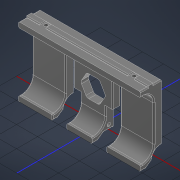
# Autodesk Inventor part: Skirt Front
Saved by Autodesk Inventor 2022.2 (Build 262287010, 287A)
## iProperties
Created: 2022-03-19
Part Number: Skirt Front
Material: ABS-Kunststoff
Document SubType Name: Modeling
Designer: sleib
Density: 1.06 g/cm^3
Appearance: Glatt - Schwarz
Author: sleib
Autodesk Inventor part; units mm, degrees
ref_plane "YZ Plane" through (0, 0, 0) normal (1, 0, 0) x (0, 1, 0)
ref_plane "XZ Plane" through (0, 0, 0) normal (0, 1, 0) x (-1, 0, 0)
ref_plane "XY Plane" through (0, 0, 0) normal (0, 0, 1) x (1, 0, 0)
sketch "Skirt" plane through (0, 0, 0) normal (0, 0, 1) x (1, 0, 0)
  line L0 (33, 20) -> (-33, 20) construction
  line L1 (-33, 20) -> (-33, 0) construction
  line L2 (-33, 0) -> (33, 0) construction
  line L3 (33, 0) -> (33, 20) construction
  line L4 (0, 20) -> (0, 0) construction
  line L5 (33, 20) -> (28, 20)
  line L6 (-33, 20) -> (-28, 20)
  line L7 (33, 20) -> (33, 13)
  line L8 (33, 0) -> (33, 7)
  line L9 (33, 13) -> (34, 13)
  line L10 (33, 7) -> (34, 7)
  line L11 (34, 7) -> (34, 13)
  line L12 (-29, 0) -> (-29, 9)
  line L13 (-29, 9) -> (-33, 14.7126)
  line L14 (-33, 20) -> (-33, 14.7126)
  line L15 (-28, 20) -> (-28, 18)
  line L16 (28, 20) -> (28, 18)
  arc A0 (17, 7) -> (28, 18) centre (17, 18) ccw
  arc A1 (-28, 18) -> (-17, 7) centre (-17, 18) ccw
  line L17 (17, 7) -> (-17, 7)
  line L18 (-29, 0) -> (33, 0)
  line L19 (33, 0.4) -> (32.6, 0)
  line L20 (-29, 0.4) -> (-28.6, 0)
  line L21 (33.2, 13) -> (34, 12.2)
  line L22 (34, 7.8002) -> (33.2, 7)
  point P0 (34, 10)
  point P1 (33, 10)
  dimension "d4" = 66
  dimension "d5" = 20
  dimension "d6" = 5
  dimension "d7" = 5
  dimension "d18" = 1
  dimension "d23" = 9
  dimension "d24" = 4
  dimension "d27" = 35
  dimension "d31" = 2
  dimension "d32" = 2
  dimension "d34" = 6
  dimension "d35" = 13
  dimension "d36" = 0.4
  dimension "d37" = 0.4
  dimension "d38" = 0.4
  dimension "d39" = 0.4
  dimension "d40" = 0.2
  dimension "d41" = 0.8
  dimension "d42" = 0.8002
  measures "d4" distance of L5.start L14.start
  measures "d5" distance of L8.start L5.start
  measures "d6" distance of L5.start L16.start
  measures "d7" distance of L14.start L15.start
  measures "d18" distance of L9.start L11.end
  measures "d23" distance of L12.start L12.end
  measures "d24" distance between parallel lines of L12 L14
  measures "d27" angle of L1 L13
  measures "d31" distance of L15.start L15.end
  measures "d32" distance of L16.start L16.end
  measures "d34" distance between parallel lines of L10 L9
  measures "d35" distance between parallel lines of L17 L0
  measures "d36" distance from line of L18 L19.start
  measures "d37" distance from line of L8 L19.end
  measures "d38" distance from line of L18 L20.start
  measures "d39" distance from line of L12 L20.end
  measures "d40" distance from line of L7 L21.start
  measures "d41" distance from line of L21.end L9
  measures "d42" distance from line of L10 L22.start
sketch "Skizze1" plane through (0, 0, 0) normal (1, 0, 0) x (0, 1, 0)
  circle A0 centre (-25, 4) radius 4 construction
  circle A1 centre (-25, 4) radius 1.7
  circle A2 centre (-25, 4) radius 3
  arc A3 (-20.4767, 0) -> (-29, 9) centre (-29.49, 0) ccw
  line L0 (33, 20) -> (-33, 20) construction
  line L1 (-33, 20) -> (-33, 0) construction
  line L2 (-33, 0) -> (33, 0) construction
  line L3 (33, 0) -> (33, 20) construction
  line L4 (0, 20) -> (0, 0) construction
  line L5 (33, 20) -> (28, 20)
  line L6 (-33, 20) -> (-28, 20)
  line L7 (33, 20) -> (33, 13)
  line L8 (33, 0) -> (33, 7)
  line L9 (33, 13) -> (34, 13)
  line L10 (33, 7) -> (34, 7)
  line L11 (34, 7) -> (34, 13)
  line L12 (-29, 0) -> (-29, 9)
  line L13 (-29, 9) -> (-33, 14.7126)
  line L14 (-33, 20) -> (-33, 14.7126)
  line L15 (-28, 20) -> (-28, 18)
  line L16 (28, 20) -> (28, 18)
  arc A4 (17, 7) -> (28, 18) centre (17, 18) ccw
  arc A5 (-28, 18) -> (-17, 7) centre (-17, 18) ccw
  line L17 (17, 7) -> (-17, 7)
  line L18 (-29, 0) -> (33, 0)
  line L19 (33, 0.4) -> (32.6, 0)
  line L20 (-29, 0.4) -> (-28.6, 0)
  line L21 (33.2, 13) -> (34, 12.2)
  line L22 (34, 7.8002) -> (33.2, 7)
  point P0 (-20.4767, 0)
  point P1 (-22.76, 5.9956)
  dimension "d43" = 8
  dimension "d44" = 3.4
  dimension "d80" = 6
  constraints: 4 centre point, 2 coincident, 2 point on circle, 1 tangent, 7 other
  measures "d43" diameter of A0
  measures "d44" diameter of A1
  measures "d80" diameter of A2
extrude "Extrusion1" add sketch "Skizze1" along normal mid plane 116 contours A3 L13 L14 L6 L15 A5 L17 A4 L16 L5 L7 L9 L21 L11 L22 L10 L8 L19 L18
sketch "Skizze2" plane through (58, 32.6, 0) normal (0, 0, -1) x (-1, 0, 0)
  line L0 (0, -65.6) -> (46, -65.6)
  line L1 (46, -65.6) -> (46, -40.6)
  line L2 (116, -65.6) -> (70, -65.6)
  line L3 (70, -65.6) -> (70, -40.6)
  line L4 (116, -65.6) -> (0, -65.6) projected
  line L5 (39.5, -40.6) -> (39.5, -15.6)
  line L6 (76.5, -40.6) -> (76.5, -15.6)
  line L7 (116, -15.6) -> (0, -15.6) projected
  line L8 (64, -22.2077) -> (70, -32.6)
  line L9 (70, -32.6) -> (64, -42.9923)
  line L10 (64, -42.9923) -> (52, -42.9923)
  line L11 (52, -42.9923) -> (46, -32.6)
  line L12 (46, -32.6) -> (52, -22.2077)
  line L13 (52, -22.2077) -> (64, -22.2077)
  line L14 (58, -15.6) -> (58, -65.6) construction
  line L15 (39.5, -40.6) -> (46, -40.6)
  line L16 (70, -40.6) -> (76.5, -40.6)
  line L17 (0, -15.6) -> (32, -15.6)
  line L18 (32, -15.6) -> (32, -65.6)
  line L19 (32, -65.6) -> (0, -65.6)
  line L20 (0, -65.6) -> (0, -15.6)
  line L21 (116, -15.6) -> (84, -15.6)
  line L22 (84, -15.6) -> (84, -65.6)
  line L23 (84, -65.6) -> (116, -65.6)
  line L24 (116, -65.6) -> (116, -15.6)
  point P0 (58, -32.6)
  point P1 (58, -32.6)
  point P2 (39.5, -15.6)
  point P3 (76.5, -15.6)
  dimension "d53" = 4
  dimension "d54" = 6.6077
  dimension "d55" = 24
  dimension "d56" = 37
  dimension "d78" = 25
  dimension "d79" = 7.5
  constraints: 46 end point, 7 horizontal, 4 parallel, 4 perpendicular, 3 point on line, 2 collinear, 2 midpoint, 1 coincident, 16 other
  measures "d53" distance from line of L1.end L11
  measures "d54" distance between parallel lines of L13 L7
  measures "d55" distance between parallel lines of L3 L1
  measures "d56" distance between parallel lines of L6 L5
  measures "d78" distance between parallel lines of L4 L15
  measures "d79" distance between parallel lines of L5 L18
extrude "Extrusion2" cut sketch "Skizze2" against normal through all contours L18 L7 L5 L15 L1 L0 | L3 L16 L6 L7 L22 L2 | L8 L9 L10 L11 L12 L13
extrude "Extrusion7" add sketch "Skizze1" along normal mid plane 24 contours A2 | A3 L18 L20 L12
fillet "Rundung1" radius 3 6 edges at (6, 10.3923, 3.5) (-6, 10.3923, 3.5) (-12, 0, 3.5) (-6, -10.3923, 3.5) (6, -10.3923, 3.5) (12, 0, 3.5)
sketch "Skizze3" plane through (58, 32.6, 0) normal (0, 0, -1) x (-1, 0, 0)
  line L0 (116, 0) -> (116, -53.0767) projected
  line L1 (116, 0) -> (0, 0) projected
  line L2 (0, -53.0767) -> (0, 0) projected
  line L3 (51.134, -41.4923) -> (46.866, -34.1) projected
  arc A0 (46.866, -31.1) -> (46.866, -34.1) centre (49.4641, -32.6) ccw projected
  line L4 (46.866, -31.1) -> (51.134, -23.7077) projected
  arc A1 (53.7321, -22.2077) -> (51.134, -23.7077) centre (53.7321, -25.2077) ccw projected
  line L5 (53.7321, -22.2077) -> (62.2679, -22.2077) projected
  arc A2 (64.866, -23.7077) -> (62.2679, -22.2077) centre (62.2679, -25.2077) ccw projected
  line L6 (64.866, -23.7077) -> (69.134, -31.1) projected
  arc A3 (69.134, -34.1) -> (69.134, -31.1) centre (66.5359, -32.6) ccw projected
  line L7 (69.134, -34.1) -> (64.866, -41.4923) projected
  arc A4 (62.2679, -42.9923) -> (64.866, -41.4923) centre (62.2679, -39.9923) ccw projected
  line L8 (62.2679, -42.9923) -> (53.7321, -42.9923) projected
  arc A5 (51.134, -41.4923) -> (53.7321, -42.9923) centre (53.7321, -39.9923) ccw projected
  line L9 (116, 1.4) -> (0, 1.4) projected
  line L10 (0, 0.6) -> (0, 1.4) projected
  line L11 (116, 0.6) -> (0, 0.6) projected
  line L12 (116, 1.4) -> (116, 0.6) projected
  circle A6 centre (45.5, -3.4) radius 2.25
  circle A7 centre (70.5, -3.4) radius 2.25
  line L13 (116, 0) -> (0, 0) projected
  line L14 (58, 0) -> (58, -61.2) construction
  line L15 (32, -53.0767) -> (32, -15.6) projected
  line L16 (32, -15.6) -> (39.5, -15.6) projected
  line L17 (39.5, -15.6) -> (39.5, -40.6) projected
  line L18 (39.5, -40.6) -> (46, -40.6) projected
  line L19 (46, -40.6) -> (46, -61.2) projected
  line L20 (70, -61.2) -> (70, -40.6) projected
  line L21 (70, -40.6) -> (76.5, -40.6) projected
  line L22 (76.5, -40.6) -> (76.5, -15.6) projected
  line L23 (76.5, -15.6) -> (84, -15.6) projected
  line L24 (84, -15.6) -> (84, -53.0767) projected
  line L25 (116, -53.0767) -> (84, -53.0767) projected
  line L26 (32, -53.0767) -> (0, -53.0767) projected
  line L27 (70, -61.2) -> (46, -61.2) projected
  point P0 (58, -32.6)
  dimension "d58" = 4.5
  dimension "d59" = 25
  dimension "d60" = 4
  constraints: 2 centre point, 2 end point, 1 equal radius, 1 horizontal alignment, 1 midpoint, 1 symmetric about line
  measures "d58" diameter of A6
  measures "d59" distance of A7.centre A6.centre
  measures "d60" distance from line of A6.centre L11
extrude "Extrusion3" cut sketch "Skizze3" against normal blind 6 contours A6 | A7
sketch "Skizze4" plane through (-58, 28, 18) normal (0, -1, 0) x (1, 0, 0)
  line L0 (0, -5.8) -> (116, -5.8) projected
  line L1 (116, -10.1998) -> (116, -5.8) projected
  line L2 (0, -10.1998) -> (116, -10.1998) projected
  line L3 (0, -5.8) -> (0, -10.1998) projected
  circle A0 centre (16, -7.9999) radius 1.7
  circle A1 centre (100, -7.9999) radius 1.7
  circle A2 centre (16, -7.9999) radius 3
  circle A3 centre (100, -7.9999) radius 3
  line L4 (0, -7.9999) -> (116, -7.9999) construction
  line L5 (0, -5.8) -> (116, -5.8) construction
  line L6 (58, -5.8) -> (58, -10.1998) construction
  line L7 (0, -10.1998) -> (116, -10.1998) construction
  point P0 (58, -18)
  dimension "d63" = 3.4
  dimension "d64" = 6
  dimension "d65" = 84
  constraints: 4 centre point, 4 end point, 4 midpoint, 2 coincident, 2 equal radius, 1 point on line, 1 symmetric about line
  measures "d63" diameter of A0
  measures "d64" diameter of A2
  measures "d65" distance of A1.centre A0.centre
extrude "Extrusion4" cut sketch "Skizze4" against normal through all contours A0 | A1
extrude "Extrusion5" cut sketch "Skizze4" along normal blind 11 and the other way blind 2 contours A2 L0 | L0 A2 L2 | L2 A2 | A3 L0 | L0 A3 L2 | L2 A3 | A0 | A1
sketch "Skizze5" plane through (-58, 33, 20) normal (0, 1, 0) x (1, 0, 0)
  circle A0 centre (16, 9.9999) radius 1.7 projected
  circle A1 centre (16, 9.9999) radius 1.7 projected
  circle A2 centre (100, 9.9999) radius 1.7 projected
  circle A3 centre (100, 9.9999) radius 1.7 projected
  line L0 (13, 6.9999) -> (19, 6.9999)
  line L1 (19, 6.9999) -> (19, 12.9999)
  line L2 (19, 12.9999) -> (13, 12.9999)
  line L3 (13, 12.9999) -> (13, 6.9999)
  line L4 (13, 6.9999) -> (19, 12.9999) construction
  line L5 (19, 6.9999) -> (13, 12.9999) construction
  line L6 (97, 6.9999) -> (103, 6.9999)
  line L7 (103, 6.9999) -> (103, 12.9999)
  line L8 (103, 12.9999) -> (97, 12.9999)
  line L9 (97, 12.9999) -> (97, 6.9999)
  line L10 (97, 6.9999) -> (103, 12.9999) construction
  line L11 (103, 6.9999) -> (97, 12.9999) construction
  point P0 (58, 20)
  dimension "d74" = 6
  dimension "d75" = 6
  constraints: 24 end point, 4 midpoint, 4 parallel, 2 equal length, 2 horizontal, 2 perpendicular
  measures "d74" distance of L2.end L1.end
  measures "d75" distance of L1.end L0.end
extrude "Extrusion6" cut sketch "Skizze5" along normal through all contours A2 | L3 L2 L1 L0 | L9 L8 L7 L6
fillet "Rundung2" radius 1 44 edges at (-58, 28, 19) (-58, 24.7782, 10.2218) (58, 28, 19) (58, 24.7782, 10.2218) (-18.5, 4.5, 7) (18.5, 4.5, 7) (-12, -24.7782, 10.2218) (-12, -28, 19) (-12, -12.5, 7) (12, -24.7782, 10.2218) (12, -28, 19) (12, -12.5, 7) (-12, -33, 17.3563) (12, -33, 17.3563) (12, -31, 11.8563) (-12, -31, 11.8563) (58, 33, 16.5) (58, 33, 3.7) (-58, 33, 16.5) (-58, 33, 3.7) (-26, -24.7782, 10.2218) (-26, -28, 19) (-26, 0, 7) (-26, -30.5, 20) (-26, -33, 17.3563) (-26, -31, 11.8563) (26, -24.7782, 10.2218) (26, -28, 19) (26, 0, 7) (26, -33, 17.3563) (26, -31, 11.8563) (-58, -24.7782, 10.2218) (-58, -28, 19) (-58, 0, 7) (58, -33, 17.3563) (58, -31, 11.8563) (-58, -33, 17.3563) (-58, -31, 11.8563) (-58, -22.9457, 6.1977) (-26, -22.9457, 6.1977) (12, -29, 4.7) (-12, -29, 4.7) (26, -22.9457, 6.1977) (58, -22.9457, 6.1977)
fillet "Rundung3" radius 1 4 edges at (-58, 32.6, 13) (-58, 32.6, 7) (58, 32.6, 13) (58, 32.6, 7)
